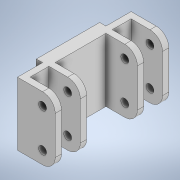
# Autodesk Inventor part: pully mount
Saved by Autodesk Inventor 2020 (Build 240168000, 168)
## iProperties
Created: 2019-09-15
Part Number: pully mount
Material: Generic
Document SubType Name: Modeling
Designer: tbloo
Density: 1 g/cm^3
Appearance: Default
Author: tbloo
Autodesk Inventor part; units mm, degrees
ref_plane "YZ Plane" through (0, 0, 0) normal (1, 0, 0) x (0, 1, 0)
ref_plane "XZ Plane" through (0, 0, 0) normal (0, 1, 0) x (-1, 0, 0)
ref_plane "XY Plane" through (0, 0, 0) normal (0, 0, 1) x (1, 0, 0)
sketch "Sketch1" plane through (0, 0, 0) normal (1, 0, 0) x (0, 1, 0)
  line L0 (0, 0) -> (32, 0)
  line L1 (32, 0) -> (32, 32)
  line L2 (32, 32) -> (0, 32)
  line L3 (0, 32) -> (0, 0)
  dimension "d0" = 32
  dimension "d1" = 32
  constraints: 8 end point, 2 parallel, 1 horizontal, 1 perpendicular
  measures "d0" distance of L2.end L1.end
  measures "d1" distance of L1.end L0.end
extrude "Extrusion1" add sketch "Sketch1" along normal blind 3.175
sketch "Sketch2" plane through (3.175, 0, 0) normal (1, 0, 0) x (0, 0, -1)
  line L0 (0, 32) -> (-32, 32) projected
  line L1 (-32, 0) -> (0, 0) projected
  line L2 (-32, 32) -> (-44.7, 32)
  line L3 (-44.7, 32) -> (-44.7, 0)
  line L4 (-44.7, 0) -> (-32, 0)
  line L5 (0, 32) -> (12.7, 32)
  line L6 (12.7, 32) -> (12.7, 0)
  line L7 (12.7, 0) -> (0, 0)
  dimension "d4" = 12.7
  dimension "d5" = 90
  dimension "d6" = 12.7
  constraints: 12 end point, 3 perpendicular, 2 horizontal
  measures "d4" distance of L0.end L2.end
  measures "d5" angle of L3 L2
  measures "d6" distance of L0.start L5.end
extrude "Extrusion2" add sketch "Sketch2" along normal blind 3.175
sketch "Sketch3" plane through (6.35, 0, 0) normal (1, 0, 0) x (0, 0, -1)
  line L0 (-32, 32) -> (-32, 0) projected
  line L1 (0, 0) -> (0, 32) projected
  line L2 (12.7, 0) -> (12.7, 32) projected
  line L3 (-44.7, 32) -> (-44.7, 0) projected
  line L4 (-32, 32) -> (-44.7, 32) projected
  line L5 (-44.7, 0) -> (-32, 0) projected
  line L6 (-44.7, 32) -> (-41.525, 32)
  line L7 (-41.525, 32) -> (-41.525, 0)
  line L8 (-41.525, 0) -> (-44.7, 0)
  line L9 (-44.7, 0) -> (-44.7, 32)
  line L10 (-32, 0) -> (0, 0) projected
  line L11 (-32, 32) -> (-28.825, 32)
  line L12 (-28.825, 32) -> (-28.825, 0)
  line L13 (-28.825, 0) -> (-32, 0)
  line L14 (-32, 0) -> (-32, 32)
  line L15 (0, 32) -> (-32, 32) projected
  line L16 (0, 32) -> (-3.175, 32)
  line L17 (-3.175, 32) -> (-3.175, 0)
  line L18 (-3.175, 0) -> (0, 0)
  line L19 (0, 0) -> (0, 32)
  line L20 (0, 0) -> (12.7, 0) projected
  line L21 (12.7, 32) -> (9.525, 32)
  line L22 (9.525, 32) -> (9.525, 0)
  line L23 (9.525, 0) -> (12.7, 0)
  line L24 (12.7, 0) -> (12.7, 32)
  dimension "d9" = 3.175
  dimension "d10" = 3.175
  dimension "d11" = 3.175
  dimension "d12" = 3.175
  constraints: 32 end point, 8 parallel, 4 horizontal, 4 perpendicular, 4 point on line
  measures "d9" distance of L7.end L8.end
  measures "d10" distance of L12.end L13.end
  measures "d11" distance of L18.end L17.end
  measures "d12" distance of L23.end L22.end
extrude "Extrusion3" add sketch "Sketch3" along normal blind 15.875 contours L11 L12 L10 L0 | L22 L21 L2 L20 | L7 L5 L3 L4 | L15 L1 L10 L17
fillet "Fillet1" radius 6.35 8 edges at (22.225, 32, 43.1125) (22.225, 32, 30.4125) (22.225, 0, 43.1125) (22.225, 0, 30.4125) (22.225, 0, 1.5875) (22.225, 32, 1.5875) (22.225, 32, -11.1125) (22.225, 0, -11.1125)
sketch "Sketch4" plane through (3.175, 0, 44.7) normal (0, 0, 1) x (1, 0, 0)
  arc A0 (19.05, 25.65) -> (12.7, 32) centre (12.7, 25.65) ccw projected
  arc A1 (12.7, 0) -> (19.05, 6.35) centre (12.7, 6.35) ccw projected
  point P0 (-3.175, 0)
  constraints: 2 coincident
hole "Hole1" at (15.875, 25.65, 44.7) at (15.875, 6.35, 44.7) direction (0, 0, -1) diameter 4 end through all
body "Solid1"
